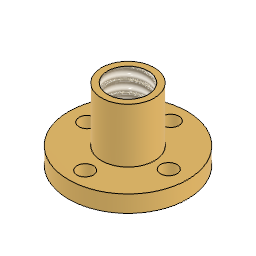
nut_housing_screw_assembly (Autodesk Fusion 360 archive; units mm, degrees)
design "Screw nut"
part number: 2026-06-28-14-14-10-628
Autodesk Fusion 360 part; units mm, degrees
sketch "Sketch1" plane through (0, 0, 0) normal (0, 0, 1) x (1, 0, 0)
  circle A0 centre (0, 0) radius 10.9
  dimension "d1" = 21.8
  constraint coincident A0.centre origin
  measures "d1" diameter of A0
extrude "Extrude1" add sketch "Sketch1" along normal blind 3.1
sketch "Sketch2" plane through (0, 0, 3.1) normal (0, 0, 1) x (-1, 0, 0)
  circle A0 centre (0, 0) radius 10.9
  circle A1 centre (0, 0) radius 4.85
  dimension "d4" = 9.7
  constraint coincident A0.centre A1.centre
  measures "d4" diameter of A1
extrude "Extrude2" add sketch "Sketch2" along normal blind 10 contours A1
sketch "Sketch3" plane through (0, 0, 0) normal (0, 0, 1) x (1, 0, 0)
  circle A0 centre (0, 0) radius 4.85
  dimension "d7" = 9.7
  constraint coincident A0.centre origin
  measures "d7" diameter of A0
extrude "Extrude3" add sketch "Sketch3" against normal blind 1.3
sketch "Sketch4" plane through (0, 0, 13.1) normal (0, 0, 1) x (-1, 0, 0)
  circle A0 centre (0, 0) radius 4.85
  circle A1 centre (0, 0) radius 3.5
  dimension "d10" = 7
  constraint concentric A0 A1
  measures "d10" diameter of A1
extrude "Extrude4" cut sketch "Sketch4" against normal through all contours A1
thread "Thread1" "ACME Screw Threads 3/8 0.3750 0.3750 4G" major diameter 9.906 minor diameter 7.4727 pitch 2.1167 angle 29 resizes the face on face at (-3.4826, 0.3485, 8.3)
sketch "Sketch5" plane through (0, 0, 3.1) normal (0, 0, 1) x (-1, 0, 0)
  circle A0 centre (0, 0) radius 4.85
  circle A1 centre (0, 0) radius 10.9
  line L0 (-10.9, 0) -> (10.9, 0) construction
  circle A2 centre (7.5, 0) radius 1.5
  circle A3 centre (7.5, 0) radius 1.5
  dimension "d14" = 3
  dimension "d18" = 3
  constraint coincident A1 L0.start
  constraint coincident A1 L0.end
  constraint horizontal L0
  constraint coincident L0 A2.centre
  measures "d14" diameter of A2
  measures "d18" diameter of A3
extrude "Extrude5" cut sketch "Sketch5" against normal through all contours A2 A3
mirror "Mirror1" about plane through (0, 0, 0) normal (1, 0, 0) of "Extrude5"
sketch "Sketch6" plane through (0, 0, 3.1) normal (0, 0, 1) x (-1, 0, 0)
  circle A0 centre (-7.5, 0) radius 1.5
  circle A1 centre (7.5, 0) radius 1.5
  circle A2 centre (0, 0) radius 4.85
  circle A3 centre (0, 0) radius 10.9
  circle A4 centre (0, -7.875) radius 1.5
  line L0 (0, -4.85) -> (0, -10.9) construction
  dimension "d19" = 3
  constraint coincident A3 L0.end
  constraint coincident A2 L0.start
  constraint midpoint A4.centre L0
  measures "d19" diameter of A4
extrude "Extrude6" cut sketch "Sketch6" against normal through all contours A4
mirror "Mirror2" about plane through (0, 0, 0) normal (0, 1, 0) of "Extrude6"
